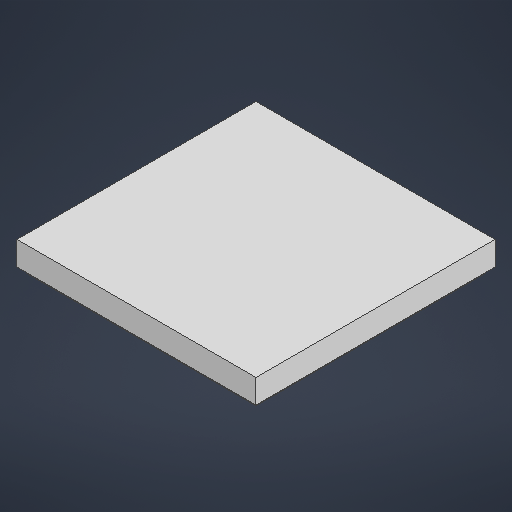
# Autodesk Inventor part: plantBottomPlate
Saved by Autodesk Inventor 2026.1 (Build 301233020, 233B)
## iProperties
Created: 2025-12-18
Part Number: plantBottomPlate
Material: Generic
Document SubType Name: Modeling
Designer: Fish
Density: 1 g/cm^3
Appearance: Default
Author: Fish
Autodesk Inventor part; units mm, degrees
ref_plane "YZ Plane" through (0, 0, 0) normal (1, 0, 0) x (0, 1, 0)
ref_plane "XZ Plane" through (0, 0, 0) normal (0, 1, 0) x (-1, 0, 0)
ref_plane "XY Plane" through (0, 0, 0) normal (0, 0, 1) x (1, 0, 0)
sketch "Sketch1" plane through (0, 0, 0) normal (0, 1, 0) x (-1, 0, 0)
  arc A0 (52.0258, 55.1946) -> (51.0258, 56.1946) centre (51.0258, 55.1946) ccw
  line L0 (-43.9742, 56.1946) -> (51.0258, 56.1946)
  arc A1 (-43.9742, 56.1946) -> (-44.9742, 55.1946) centre (-43.9742, 55.1946) ccw
  line L1 (-44.9742, -39.8054) -> (-44.9742, 55.1946)
  arc A2 (-44.9742, -39.8054) -> (-43.9742, -40.8054) centre (-43.9742, -39.8054) ccw
  line L2 (51.0258, -40.8054) -> (-43.9742, -40.8054)
  arc A3 (51.0258, -40.8054) -> (52.0258, -39.8054) centre (51.0258, -39.8054) ccw
  line L3 (52.0258, 55.1946) -> (52.0258, -39.8054)
  line L4 (-11.2742, 54.1946) -> (-42.9742, 54.1946)
  line L5 (-11.2742, -38.8054) -> (-11.2742, 54.1946)
  line L6 (-42.9742, -38.8054) -> (-11.2742, -38.8054)
  line L7 (-42.9742, 54.1946) -> (-42.9742, -38.8054)
  line L8 (50.0258, -38.8054) -> (50.0258, 54.1946)
  line L9 (-9.2742, -38.8054) -> (50.0258, -38.8054)
  line L10 (-9.2742, 54.1946) -> (-9.2742, -38.8054)
  line L11 (50.0258, 54.1946) -> (-9.2742, 54.1946)
  line L12 (53.5258, 57.6946) -> (-46.4742, 57.6946)
  line L13 (-46.4742, 57.6946) -> (-46.4742, -42.3054)
  line L14 (-46.4742, -42.3054) -> (53.5258, -42.3054)
  line L15 (53.5258, -42.3054) -> (53.5258, 57.6946)
  line L16 (51.0258, 55.1946) -> (-43.9742, 55.1946) construction
  line L17 (-43.9742, 55.1946) -> (-43.9742, -39.8054) construction
  line L18 (-43.9742, -39.8054) -> (51.0258, -39.8054) construction
  line L19 (51.0258, -39.8054) -> (51.0258, 55.1946) construction
  line L20 (-41.4742, -37.3054) -> (-12.7742, -37.3054)
  line L21 (-12.7742, -37.3054) -> (-12.7742, 52.6946)
  line L22 (-12.7742, 52.6946) -> (-41.4742, 52.6946)
  line L23 (-41.4742, 52.6946) -> (-41.4742, -37.3054)
  line L24 (-7.7742, -37.3054) -> (48.5258, -37.3054)
  line L25 (48.5258, -37.3054) -> (48.5258, 52.6946)
  line L26 (48.5258, 52.6946) -> (-7.7742, 52.6946)
  line L27 (-7.7742, 52.6946) -> (-7.7742, -37.3054)
  line L28 (-10.2742, 55.1946) -> (-10.2742, -39.8054) construction
  arc A4 (51.0258, -40.6054) -> (51.8258, -39.8054) centre (51.0258, -39.8054) ccw
  line L29 (51.0258, -40.6054) -> (-43.9742, -40.6054)
  arc A5 (-44.7742, -39.8054) -> (-43.9742, -40.6054) centre (-43.9742, -39.8054) ccw
  line L30 (-44.7742, -39.8054) -> (-44.7742, 55.1946)
  arc A6 (-43.9742, 55.9946) -> (-44.7742, 55.1946) centre (-43.9742, 55.1946) ccw
  line L31 (-43.9742, 55.9946) -> (51.0258, 55.9946)
  arc A7 (51.8258, 55.1946) -> (51.0258, 55.9946) centre (51.0258, 55.1946) ccw
  line L32 (51.8258, 55.1946) -> (51.8258, -39.8054)
  line L33 (50.2258, 54.3946) -> (50.2258, -39.0054)
  line L34 (50.2258, -39.0054) -> (-9.4742, -39.0054)
  line L35 (-9.4742, -39.0054) -> (-9.4742, 54.3946)
  line L36 (-9.4742, 54.3946) -> (50.2258, 54.3946)
  line L37 (-43.1742, -39.0054) -> (-11.0742, -39.0054)
  line L38 (-11.0742, -39.0054) -> (-11.0742, 54.3946)
  line L39 (-11.0742, 54.3946) -> (-43.1742, 54.3946)
  line L40 (-43.1742, 54.3946) -> (-43.1742, -39.0054)
  point P0 (0, 0)
  point P1 (-29.6242, 39.9946)
  dimension "d0" = 2
  dimension "d1" = 2.5
  dimension "d2" = 2.5
  dimension "d3" = 2.5
  dimension "d4" = 2.5
  dimension "d5" = 2.5
  dimension "d6" = 2.5
  dimension "d7" = 2.5
  dimension "d8" = 2.5
  dimension "d9" = 5
  dimension "d10" = 1
  dimension "d11" = 2
  dimension "d12" = 2.5
  dimension "d13" = 0.2
  dimension "d14" = 0.2
  dimension "d15" = 0.2
  constraints: 82 end point, 16 point on circle, 9 horizontal, 8 centre point, 8 parallel, 6 perpendicular, 6 vertical, 4 point on line, 39 other
  measures "d0" distance between parallel lines of L3 L8
  measures "d1" distance between parallel lines of L12 L16
  measures "d2" distance between parallel lines of L15 L19
  measures "d3" distance between parallel lines of L14 L18
  measures "d4" distance between parallel lines of L13 L17
  measures "d5" distance between parallel lines of L25 L19
  measures "d6" distance between parallel lines of L16 L26
  measures "d7" distance between parallel lines of L17 L23
  measures "d8" distance between parallel lines of L18 L20
  measures "d9" distance between parallel lines of L27 L21
  measures "d10" distance between parallel lines of L10 L28
  measures "d11" distance between parallel lines of L5 L10
  measures "d12" distance between parallel lines of L21 L28
  measures "d13" distance between parallel lines of L3 L32
  measures "d14" distance between parallel lines of L8 L33
  measures "d15" distance between parallel lines of L7 L40
extrude "Extrusion1" add sketch "Sketch1" along normal blind 5 contours L3 A3 L2 A2 L1 A1 L0 A0 | L5 L6 L7 L4 | L9 L10 L11 L8 | L15 L14 L13 L12 | L23 L22 L21 L20 | L27 L26 L25 L24 | L29 A5 L30 A6 L31 A7 L32 A4 | L33 L34 L35 L36 | L40 L39 L38 L37
extrude "Extrusion2" add sketch "Sketch1" against normal blind 5 contours L3 A3 L2 A2 L1 A1 L0 A0 | L5 L6 L7 L4 | L9 L10 L11 L8 | L15 L14 L13 L12 | L29 A5 L30 A6 L31 A7 L32 A4 | L33 L34 L35 L36 | L40 L39 L38 L37
extrude "Extrusion3" add sketch "Sketch1" against normal blind 7 contours L29 A5 L30 A6 L31 A7 L32 A4
equation "\"d2\" = d1"
equation "\"d3\" = d2"
equation "\"d4\" = d1"
equation "\"d5\" = d2"
equation "\"d6\" = d1"
equation "\"d7\" = d4"
equation "\"d8\" = d7"
equation "\"d10\" = 0.5 * d11"
equation "\"d12\" = 0.5 * d9"
equation "\"d14\" = d13"
equation "\"d15\" = d14"
body "Solid1"
